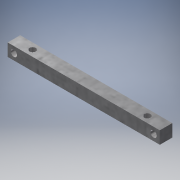
# Autodesk Inventor part: transverse
Saved by Autodesk Inventor 2016 (Build 200138000, 138)
## iProperties
Created: 2015-10-11
Part Number: transverse
Material: Aluminum
Document SubType Name: Modeling
Designer: Artur
Density: 2.7 g/cm^3
Appearance: Galvanized
Mass: 20.9124 g
Surface Area: 18.48 cm^2
Volume: 2.664 cm^3
Author: Artur
Autodesk Inventor part; units mm, degrees
ref_plane "YZ Plane" through (0, 0, 0) normal (1, 0, 0) x (0, 1, 0)
ref_plane "XZ Plane" through (0, 0, 0) normal (0, 1, 0) x (-1, 0, 0)
ref_plane "XY Plane" through (0, 0, 0) normal (0, 0, 1) x (1, 0, 0)
sketch "Sketch1" plane through (0, 0, 0) normal (1, 0, 0) x (0, 1, 0)
  line L0 (0, 0) -> (6, 0)
  line L1 (6, 0) -> (6, -6)
  line L2 (6, -6) -> (0, -6)
  line L3 (0, -6) -> (0, 0)
  dimension "d0" = 6
  dimension "d1" = 6
  constraints: 8 end point, 2 parallel, 1 horizontal, 1 perpendicular
  measures "d0" distance of L1.end L2.end
  measures "d1" distance of L2.end L0.start
extrude "Extrusion1" add sketch "Sketch1" along normal blind 73
sketch "Sketch2" plane through (0, 6, 0) normal (0, 1, 0) x (1, 0, 0)
  line L0 (0, 6) -> (73, 6) construction
  line L1 (36.5, 6) -> (36.5, 0)
  line L2 (0, 0) -> (73, 0) construction
  line L3 (0, 6) -> (0, 0) construction
  line L4 (0, 3) -> (73, 3)
  line L5 (73, 0) -> (73, 6) construction
  point P0 (3, 3)
  point P1 (70, 3)
  dimension "d8" = 3
  constraints: 4 end point, 4 midpoint, 1 point on line, 1 symmetric about line
  measures "d8" distance from line of L3 point (3, 3)
hole "Hole1" at (3, 6, -3) at (70, 6, -3) direction (0, -1, 0) diameter 3 end through all
sketch "Sketch3" plane through (0, 0, -6) normal (0, 0, -1) x (-1, 0, 0)
  line L0 (0, 6) -> (0, 0) construction
  line L1 (0, 6) -> (-73, 6) construction
  line L2 (-73, 0) -> (-73, 6) construction
  line L3 (0, 0) -> (-73, 0) construction
  line L4 (0, 3) -> (-73, 3) construction
  line L5 (0, 6) -> (-73, 6) construction
  line L6 (-36.5, 6) -> (-36.5, 0) construction
  line L7 (0, 0) -> (-73, 0) construction
  point P0 (-9, 3)
  point P1 (-64, 3)
  dimension "d16" = 9
  constraints: 4 end point, 4 midpoint, 1 point on line, 1 symmetric about line
  measures "d16" distance from line of L0 point (-9, 3)
hole "Hole2" at (9, 3, -6) at (64, 3, -6) direction (0, 0, 1) diameter 3 end through all
equation "\"d1\" = d0"
body "Solid1"
